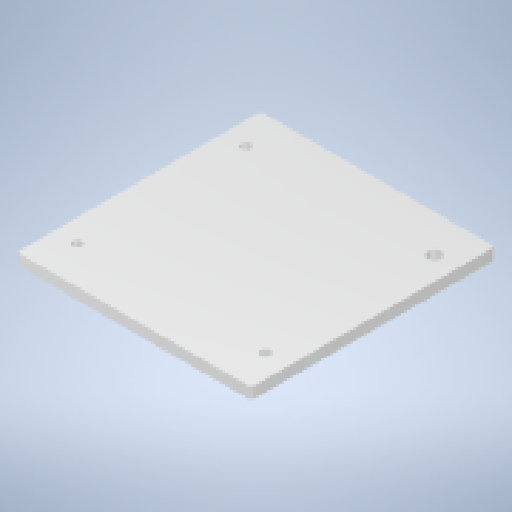
# Autodesk Inventor part: C beam gantry (small side y axis)
Saved by Autodesk Inventor 2023.2 (Build 272271000, 271)
## iProperties
Created: 2023-03-20
Part Number: C beam gantry (small side y axis)
Material: Aluminum 6061
Document SubType Name: Modeling
Designer: dmargari
Density: 2.7 g/cm^3
Appearance: Aluminum - Flat
Author: dmargari
Autodesk Inventor part; units mm, degrees
ref_plane "YZ Plane" through (0, 0, 0) normal (1, 0, 0) x (0, 1, 0)
ref_plane "XZ Plane" through (0, 0, 0) normal (0, 1, 0) x (-1, 0, 0)
ref_plane "XY Plane" through (0, 0, 0) normal (0, 0, 1) x (1, 0, 0)
sketch "Sketch1" plane through (0, 0, 0) normal (0, 1, 0) x (-1, 0, 0)
  line L0 (163.0343, -138.5167) -> (38.0343, -138.5167)
  line L1 (38.0343, -138.5167) -> (38.0343, -268.5167)
  line L2 (38.0343, -268.5167) -> (163.0343, -268.5167)
  line L3 (163.0343, -268.5167) -> (163.0343, -138.5167)
  line L4 (150.7343, -138.5167) -> (150.7343, -268.5167) construction
  line L5 (50.3343, -138.5167) -> (50.3343, -268.5167) construction
  circle A0 centre (150.7343, -158.5167) radius 2.55
  circle A1 centre (150.7343, -248.5167) radius 2.55
  circle A2 centre (50.3343, -158.5167) radius 2.55
  circle A3 centre (50.3343, -248.5167) radius 3.55
  point P0 (0, 0)
  dimension "d0" = 125
  dimension "d1" = 130
  dimension "d4" = 5.1
  dimension "d5" = 5.1
  dimension "d6" = 5.1
  dimension "d7" = 7.1
  dimension "d11" = 100.4
  dimension "d12" = 20
  dimension "d13" = 20
  dimension "d14" = 20
  dimension "d15" = 20
  constraints: 12 end point, 8 point on line, 4 centre point, 3 perpendicular, 2 parallel, 1 horizontal
  measures "d0" distance of L2.end L1.end
  measures "d1" distance of L1.end L0.end
  measures "d4" diameter of A0
  measures "d5" diameter of A1
  measures "d6" diameter of A2
  measures "d7" diameter of A3
  measures "d11" distance between parallel lines of L4 L5
  measures "d12" distance from line of L2 A1.centre
  measures "d13" distance from line of L2 A3.centre
  measures "d14" distance from line of L0 A0.centre
  measures "d15" distance from line of L0 A2.centre
extrude "Extrusion1" add sketch "Sketch1" along normal blind 6
fillet "Fillet1" radius 2 4 edges at (-163.0343, 3, -268.5167) (-163.0343, 3, -138.5167) (-38.0343, 3, -138.5167) (-38.0343, 3, -268.5167)
body "Solid1"
